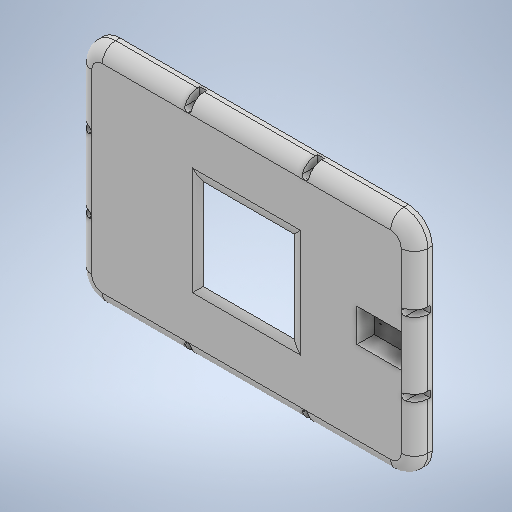
# Autodesk Inventor part: up
Saved by Autodesk Inventor 2025 (Build 290162000, 162)
## iProperties
Created: 2025-10-21
Part Number: up
Material: Generic
Document SubType Name: Modeling
Designer: hp
Density: 1 g/cm^3
Appearance: Default
Author: hp
Autodesk Inventor part; units mm, degrees
ref_plane "YZ Plane" through (0, 0, 0) normal (1, 0, 0) x (0, 1, 0)
ref_plane "XZ Plane" through (0, 0, 0) normal (0, 1, 0) x (-1, 0, 0)
ref_plane "XY Plane" through (0, 0, 0) normal (0, 0, 1) x (1, 0, 0)
sketch "Sketch1" plane through (0, 0, 0) normal (0, 0, 1) x (1, 0, 0)
  line L0 (-325, 254) -> (325, 254)
  line L1 (379, 200) -> (379, -200)
  line L2 (325, -254) -> (-325, -254)
  line L3 (-379, -200) -> (-379, 200)
  line L4 (-379, 254) -> (379, -254) construction
  line L5 (379, 254) -> (-379, -254) construction
  arc A0 (-325, 254) -> (-379, 200) centre (-325, 200) ccw
  arc A1 (379, 200) -> (325, 254) centre (325, 200) ccw
  arc A2 (325, -254) -> (379, -200) centre (325, -200) ccw
  arc A3 (-379, -200) -> (-325, -254) centre (-325, -200) ccw
  point P0 (0, 0)
  dimension "d0" = 758
  dimension "d1" = 508
  dimension "d2" = 54
  constraints: 12 end point, 8 point on circle, 8 point on line, 8 tangent, 4 centre point, 3 equal radius, 2 midpoint, 2 parallel, 1 horizontal, 1 perpendicular
  measures "d0" distance of L4.end L5.end
  measures "d1" distance of L5.start L4.end
  measures "d2" radius of A0
extrude "Extrusion1" add sketch "Sketch1" along normal blind 40
fillet "Fillet1" radius 30 8 edges at (-363.1838, 238.1838, 40) (-379, 0, 40) (-363.1838, -238.1838, 40) (0, -254, 40) (363.1838, -238.1838, 40) (379, 0, 40) (363.1838, 238.1838, 40) (0, 254, 40)
sketch "Sketch2" plane through (0, 0, 0) normal (0, 0, -1) x (-1, 0, 0)
  line L0 (289, 224) -> (-289, 224)
  line L1 (-349, 164) -> (-349, -164)
  line L2 (-289, -224) -> (289, -224)
  line L3 (349, -164) -> (349, 164)
  line L4 (349, 224) -> (-349, -224) construction
  line L5 (-349, 224) -> (349, -224) construction
  arc A0 (349, 164) -> (289, 224) centre (289, 164) ccw
  arc A1 (289, -224) -> (349, -164) centre (289, -164) ccw
  arc A2 (-349, -164) -> (-289, -224) centre (-289, -164) ccw
  arc A3 (-289, 224) -> (-349, 164) centre (-289, 164) ccw
  point P0 (0, 0)
  dimension "d6" = 698
  dimension "d7" = 448
  dimension "d8" = 60
  constraints: 12 end point, 8 point on circle, 8 point on line, 8 tangent, 4 centre point, 3 equal radius, 2 midpoint, 2 parallel, 1 horizontal, 1 perpendicular
  measures "d6" distance of L5.end L4.end
  measures "d7" distance of L5.end L4.start
  measures "d8" radius of A0
extrude "Extrusion2" cut sketch "Sketch2" against normal blind 35
sketch "Sketch3" plane through (0, 0, 40) normal (0, 0, 1) x (1, 0, 0)
  line L0 (-377.7666, 254) -> (272.2334, 254)
  line L1 (-140, 254) -> (-125, 254)
  line L2 (-125, -254) -> (-140, -254)
  line L3 (125, 254) -> (140, 254)
  line L4 (140, -254) -> (125, -254)
  line L5 (-379, -196) -> (-379, 204)
  line L6 (379, 86) -> (379, 71)
  line L7 (-379, 71) -> (-379, 86)
  line L8 (379, 224.0745) -> (379, -175.9255)
  line L9 (379, -79) -> (379, -94)
  line L10 (264.2334, -254) -> (-385.7666, -254)
  line L11 (125, 232.5) -> (125, 254)
  line L12 (140, 254) -> (140, 232.5)
  line L13 (-125, 254) -> (-125, 232.5)
  line L14 (-140, 232.5) -> (-140, 254)
  line L15 (-379, 86) -> (-357.5, 86)
  line L16 (-357.5, 71) -> (-379, 71)
  line L17 (-379, -79) -> (-357.5, -79)
  line L18 (-357.5, -94) -> (-435.7666, -94)
  line L19 (-140, -254) -> (-140, -232.5)
  line L20 (-125, -232.5) -> (-125, -254)
  line L21 (140, -232.5) -> (140, -254)
  line L22 (125, -254) -> (125, -232.5)
  line L23 (357.5, -79) -> (379, -79)
  line L24 (379, -94) -> (357.5, -94)
  line L25 (357.5, 86) -> (379, 86)
  line L26 (379, 71) -> (357.5, 71)
  arc A0 (-140, 232.5) -> (-125, 232.5) centre (-132.5, 232.5) ccw
  arc A1 (125, 232.5) -> (140, 232.5) centre (132.5, 232.5) ccw
  arc A2 (-357.5, 71) -> (-357.5, 86) centre (-357.5, 78.5) ccw
  arc A3 (-357.5, -94) -> (-357.5, -79) centre (-357.5, -86.5) ccw
  arc A4 (-125, -232.5) -> (-140, -232.5) centre (-132.5, -232.5) ccw
  arc A5 (140, -232.5) -> (125, -232.5) centre (132.5, -232.5) ccw
  arc A6 (357.5, -79) -> (357.5, -94) centre (357.5, -86.5) ccw
  arc A7 (357.5, 86) -> (357.5, 71) centre (357.5, 78.5) ccw
  circle A8 centre (132.5, 232.5) radius 2.5
  circle A9 centre (-132.5, 232.5) radius 2.5
  circle A10 centre (-357.5, 78.5) radius 2.5
  circle A11 centre (-357.5, -86.5) radius 2.5
  circle A12 centre (-132.5, -232.5) radius 2.5
  circle A13 centre (132.5, -232.5) radius 2.5
  circle A14 centre (357.5, -86.5) radius 2.5
  circle A15 centre (357.5, 78.5) radius 2.5
  line L27 (325, 254) -> (-325, 254) projected
  line L28 (-325, -254) -> (325, -254) projected
  line L29 (379, -200) -> (379, 200) projected
  line L30 (-379, 200) -> (-379, -200) projected
  line L31 (-102.5, -102.5) -> (102.5, -102.5)
  line L32 (102.5, -102.5) -> (102.5, 102.5)
  line L33 (102.5, 102.5) -> (-102.5, 102.5)
  line L34 (-102.5, 102.5) -> (-102.5, -102.5)
  line L35 (-102.5, -102.5) -> (102.5, 102.5) construction
  line L36 (102.5, -102.5) -> (-102.5, 102.5) construction
  point P0 (0, 0)
  point P1 (-132.5, -254)
  point P2 (132.5, -254)
  point P3 (-423.2666, 71)
  point P4 (301.7334, -79)
  point P5 (301.7334, 71)
  point P6 (301.7334, -94)
  point P7 (125, -163.4255)
  point P8 (-140, -163.4255)
  point P9 (-379, 78.5)
  point P10 (-132.5, -225)
  point P11 (379, -86.5)
  point P12 (-379, -94)
  dimension "d11" = 758
  dimension "d12" = 15
  dimension "d13" = 0
  dimension "d14" = 250
  dimension "d15" = 239
  dimension "d16" = 15
  dimension "d17" = 15
  dimension "d18" = 150
  dimension "d19" = 160
  dimension "d20" = 15
  dimension "d21" = 150
  dimension "d22" = 160
  dimension "d23" = 15
  dimension "d24" = 15
  dimension "d25" = 254
  dimension "d26" = 250
  dimension "d27" = 15
  dimension "d28" = 5
  dimension "d29" = 5
  dimension "d30" = 5
  dimension "d31" = 5
  dimension "d32" = 5
  dimension "d33" = 5
  dimension "d34" = 5
  dimension "d35" = 5
  dimension "d36" = 21.5
  dimension "d37" = 21.5
  dimension "d38" = 21.5
  dimension "d39" = 15
  dimension "d40" = 21.5
  dimension "d41" = 21.5
  dimension "d42" = 29
  dimension "d43" = 21.5
  dimension "d44" = 21.5
  dimension "d83" = 205
  dimension "d84" = 205
  dimension "d87" = 150
  constraints: 66 end point, 21 parallel, 17 point on circle, 16 centre point, 16 tangent, 12 point on line, 9 perpendicular, 8 coincident, 7 horizontal, 6 midpoint, 5 collinear
  measures "d11" distance of L15.start L6.start
  measures "d12" distance of L6.start L6.end
  measures "d13" distance from line of L10 point (-132.5, -254)
  measures "d14" distance from line of L3.start L13
  measures "d15" distance between parallel lines of L8 L12
  measures "d16" distance from line of L3.end L11
  measures "d17" distance between parallel lines of L16 L15
  measures "d18" distance from line of L17 point (-423.267, 71)
  measures "d19" distance between parallel lines of L10 L18
  measures "d20" distance between parallel lines of L18 L17
  measures "d21" distance of point (301.733, -79) point (301.733, 71)
  measures "d22" distance from line of L10 point (301.733, -94)
  measures "d23" distance between parallel lines of L24 L23
  measures "d24" distance from line of point (125, -163.426) L21
  measures "d25" distance from line of L8 point (125, -163.426)
  measures "d26" distance between parallel lines of L22 L20
  measures "d27" distance from line of L20 point (-140, -163.426)
  measures "d28" diameter of A8
  measures "d29" diameter of A9
  measures "d30" diameter of A10
  measures "d31" diameter of A11
  measures "d32" diameter of A12
  measures "d33" diameter of A13
  measures "d34" diameter of A14
  measures "d35" diameter of A15
  measures "d36" distance from line of L4 A5.centre
  measures "d37" distance from line of A1.centre L3
  measures "d38" distance from line of A0.centre L0
  measures "d39" distance between parallel lines of L13 L14
  measures "d40" distance of point (-379, 78.5) A2.centre
  measures "d41" distance from line of L5 A3.centre
  measures "d42" distance from line of L10 point (-132.5, -225)
  measures "d43" distance of point (379, -86.5) A6.centre
  measures "d44" distance from line of A7.centre L6
  measures "d83" distance of L33.end L32.end
  measures "d84" distance of L32.end L31.end
  measures "d87" distance between parallel lines of L23 L26
sketch "Sketch4" plane through (0, 0, 0) normal (0, 0, -1) x (-1, 0, 0)
  line L0 (-329.5439, 254) -> (320.4561, 254)
  line L1 (-140, 254) -> (-125, 254)
  line L2 (-125, -254) -> (-140, -254)
  line L3 (125, 254) -> (140, 254)
  line L4 (140, -254) -> (125, -254)
  line L5 (-379, -204) -> (-379, 196)
  line L6 (379, 86) -> (379, 71)
  line L7 (-379, 71) -> (-379, 86)
  line L8 (379, 206.0747) -> (379, -193.9253)
  line L9 (379, -79) -> (379, -94)
  line L10 (328.4561, -254) -> (-321.5439, -254)
  line L11 (125, 232.5) -> (125, 254)
  line L12 (140, 254) -> (140, 232.5)
  line L13 (-125, 254) -> (-125, 232.5)
  line L14 (-140, 232.5) -> (-140, 254)
  line L15 (-379, 86) -> (-357.5, 86)
  line L16 (-357.5, 71) -> (-379, 71)
  line L17 (-379, -79) -> (-357.5, -79)
  line L18 (-357.5, -94) -> (-371.5439, -94)
  line L19 (-140, -254) -> (-140, -232.5)
  line L20 (-125, -232.5) -> (-125, -254)
  line L21 (140, -232.5) -> (140, -254)
  line L22 (125, -254) -> (125, -232.5)
  line L23 (357.5, -79) -> (379, -79)
  line L24 (379, -94) -> (357.5, -94)
  line L25 (357.5, 86) -> (379, 86)
  line L26 (379, 71) -> (357.5, 71)
  arc A0 (-140, 232.5) -> (-125, 232.5) centre (-132.5, 232.5) ccw
  arc A1 (125, 232.5) -> (140, 232.5) centre (132.5, 232.5) ccw
  arc A2 (-357.5, 71) -> (-357.5, 86) centre (-357.5, 78.5) ccw
  arc A3 (-357.5, -94) -> (-357.5, -79) centre (-357.5, -86.5) ccw
  arc A4 (-125, -232.5) -> (-140, -232.5) centre (-132.5, -232.5) ccw
  arc A5 (140, -232.5) -> (125, -232.5) centre (132.5, -232.5) ccw
  arc A6 (357.5, -79) -> (357.5, -94) centre (357.5, -86.5) ccw
  arc A7 (357.5, 86) -> (357.5, 71) centre (357.5, 78.5) ccw
  circle A8 centre (132.5, 232.5) radius 2.5
  circle A9 centre (-132.5, 232.5) radius 2.5
  circle A10 centre (-357.5, 78.5) radius 2.5
  circle A11 centre (-357.5, -86.5) radius 2.5
  circle A12 centre (-132.5, -232.5) radius 2.5
  circle A13 centre (132.5, -232.5) radius 2.5
  circle A14 centre (357.5, -86.5) radius 2.5
  circle A15 centre (357.5, 78.5) radius 2.5
  line L27 (325, -254) -> (-325, -254) projected
  line L28 (379, 200) -> (379, -200) projected
  line L29 (-379, -200) -> (-379, 200) projected
  line L30 (-325, 254) -> (325, 254) projected
  point P0 (0, 0)
  point P1 (-132.5, -254)
  point P2 (132.5, -254)
  point P3 (-359.0439, 71)
  point P4 (365.9561, -79)
  point P5 (365.9561, 71)
  point P6 (365.9561, -94)
  point P7 (125, -181.4253)
  point P8 (-140, -181.4253)
  point P9 (-379, 78.5)
  point P10 (-132.5, -225)
  point P11 (379, -86.5)
  dimension "d45" = 758
  dimension "d46" = 15
  dimension "d47" = 0
  dimension "d48" = 250
  dimension "d49" = 239
  dimension "d50" = 15
  dimension "d51" = 15
  dimension "d52" = 150
  dimension "d53" = 160
  dimension "d54" = 15
  dimension "d55" = 150
  dimension "d56" = 160
  dimension "d57" = 15
  dimension "d58" = 15
  dimension "d59" = 254
  dimension "d60" = 250
  dimension "d61" = 15
  dimension "d62" = 5
  dimension "d63" = 5
  dimension "d64" = 5
  dimension "d65" = 5
  dimension "d66" = 5
  dimension "d67" = 5
  dimension "d68" = 5
  dimension "d69" = 5
  dimension "d70" = 21.5
  dimension "d71" = 21.5
  dimension "d72" = 21.5
  dimension "d73" = 15
  dimension "d74" = 21.5
  dimension "d75" = 21.5
  dimension "d76" = 29
  dimension "d77" = 21.5
  dimension "d78" = 21.5
  constraints: 54 end point, 19 parallel, 17 point on circle, 16 centre point, 16 tangent, 12 point on line, 8 coincident, 8 perpendicular, 6 horizontal, 5 collinear, 4 midpoint
  measures "d45" distance of L15.start L25.end
  measures "d46" distance of L25.end L6.end
  measures "d47" distance from line of L10 point (-132.5, -254)
  measures "d48" distance from line of L3.start L13
  measures "d49" distance between parallel lines of L8 L12
  measures "d50" distance from line of L12.start L11
  measures "d51" distance between parallel lines of L16 L15
  measures "d52" distance from line of L17 point (-359.044, 71)
  measures "d53" distance between parallel lines of L10 L18
  measures "d54" distance between parallel lines of L18 L17
  measures "d55" distance of point (365.956, -79) point (365.956, 71)
  measures "d56" distance from line of L10 point (365.956, -94)
  measures "d57" distance between parallel lines of L24 L23
  measures "d58" distance from line of point (125, -181.425) L21
  measures "d59" distance from line of L8 point (125, -181.425)
  measures "d60" distance between parallel lines of L22 L20
  measures "d61" distance from line of L20 point (-140, -181.425)
  measures "d62" diameter of A8
  measures "d63" diameter of A9
  measures "d64" diameter of A10
  measures "d65" diameter of A11
  measures "d66" diameter of A12
  measures "d67" diameter of A13
  measures "d68" diameter of A14
  measures "d69" diameter of A15
  measures "d70" distance from line of L4 A5.centre
  measures "d71" distance from line of A1.centre L3
  measures "d72" distance from line of A0.centre L0
  measures "d73" distance between parallel lines of L13 L14
  measures "d74" distance of point (-379, 78.5) A2.centre
  measures "d75" distance from line of L5 A3.centre
  measures "d76" distance from line of L10 point (-132.5, -225)
  measures "d77" distance of point (379, -86.5) A6.centre
  measures "d78" distance from line of A7.centre L6
extrude "Extrusion3" cut sketch "Sketch3" against normal blind 35 contours L0 L13 A0 L14 | L0 L12 A1 L11 | L2 L19 A4 L20 | L4 L22 A5 L21 | L5 L15 A2 L16 | L5 L17 A3 L18 | L6 L26 A7 L25 | L8 L24 A6 L23 | A13
extrude "Extrusion4" cut sketch "Sketch3" against normal through all contours A8 | A9 | A10 | A11 | A12 | A13 | A14 | A15
extrude "Extrusion5" cut sketch "Sketch3" against normal blind 10 contours L34 L33 L32 L31
fillet "Fillet2" radius 40 4 edges at (102.5, 0, 40) (0, -102.5, 40) (-102.5, 0, 40) (0, 102.5, 40)
sketch "Sketch6" plane through (0, 0, 40) normal (0, 0, 1) x (1, 0, 0)
  line L0 (-325, 224) -> (325, 224) projected
  line L1 (283.7823, 13.3743) -> (328.5995, 13.3743)
  line L2 (337.9658, 20.6774) -> (276.5853, 20.6774)
  line L3 (337.9658, 20.6774) -> (276.5853, 20.6774)
  arc A0 (339.1694, 33.055) -> (273.3647, 25.3501) centre (315.2399, -47.431) ccw
  arc A1 (339.1694, 33.055) -> (273.3647, 25.3501) centre (315.2399, -47.431) ccw
  arc A2 (336.6026, 29.0932) -> (276.5202, 21.4818) centre (315.2559, -43.3443) ccw
  arc A3 (336.6026, 29.0932) -> (276.5202, 21.4818) centre (315.2559, -43.3443) ccw
  line L4 (283.7823, 13.3743) -> (328.5995, 13.3743)
  line L5 (337.9658, -19.3226) -> (337.9658, -23.873)
  line L6 (337.9658, 25.2279) -> (337.9658, 20.6774)
  line L7 (337.9658, 25.2279) -> (337.9658, 20.6774)
  line L8 (337.9658, -19.3226) -> (337.9658, -23.873)
  arc A4 (336.6026, 29.0932) -> (337.9658, 25.2279) centre (341.5853, 28.6774) ccw
  arc A5 (337.9658, 25.2279) -> (345.8797, 26.1166) centre (341.5853, 28.6774) ccw
  circle A6 centre (341.5853, 28.6774) radius 2.6
  arc A7 (345.8455, -24.7052) -> (345.8797, 26.1166) centre (244.5247, 0.7738) ccw
  line L9 (328.5995, 13.3743) -> (328.5995, -11.7233)
  line L10 (283.7823, -11.7233) -> (283.7823, 13.3743)
  line L11 (328.5995, 13.3743) -> (328.5995, -11.7233)
  arc A8 (266.5894, 20.4761) -> (266.5894, -19.1212) centre (270.1885, 0.6774) ccw
  line L12 (328.5995, -11.7233) -> (283.7823, -11.7233)
  line L13 (328.5995, -11.7233) -> (283.7823, -11.7233)
  line L14 (276.5853, -19.3226) -> (337.9658, -19.3226)
  line L15 (276.5853, -19.3226) -> (337.9658, -19.3226)
  arc A9 (276.5439, -19.9643) -> (336.5926, -27.592) centre (318.3549, 69.0112) ccw
  arc A10 (276.5439, -19.9643) -> (336.5926, -27.592) centre (318.3549, 69.0112) ccw
  arc A11 (273.3471, -24.0019) -> (339.2228, -31.7292) centre (315.1175, 47.4314) ccw
  arc A12 (273.3471, -24.0019) -> (339.2228, -31.7292) centre (315.1175, 47.4314) ccw
  circle A13 centre (341.5853, 28.6774) radius 2.6
  circle A14 centre (343.2402, 16.9907) radius 1.5
  arc A15 (345.8797, 26.1166) -> (339.1694, 33.055) centre (341.5853, 28.6774) ccw
  circle A16 centre (343.2402, 16.9907) radius 1.5
  circle A17 centre (343.5969, -11.7233) radius 1.5
  circle A18 centre (341.5853, -27.3226) radius 2.6
  circle A19 centre (341.5853, -27.3226) radius 2.6
  circle A20 centre (263.5183, -9.7117) radius 1.5
  circle A21 centre (263.5183, -9.7117) radius 1.5
  circle A22 centre (264.1372, 12.2943) radius 1.5
  circle A23 centre (264.1372, 12.2943) radius 1.5
  circle A24 centre (271.5853, 20.6774) radius 2.6
  line L16 (283.7823, -11.7233) -> (283.7823, 13.3743)
  circle A25 centre (271.5853, 20.6774) radius 2.6
  circle A26 centre (271.5853, -19.3226) radius 2.6
  circle A27 centre (271.5853, -19.3226) radius 2.6
  arc A28 (266.5894, 20.4761) -> (266.5894, -19.1212) centre (270.1885, 0.6774) ccw
  arc A29 (339.1694, 33.055) -> (336.6026, 29.0932) centre (341.5853, 28.6774) ccw
  arc A30 (345.8455, -24.7052) -> (345.8797, 26.1166) centre (244.5247, 0.7738) ccw
  circle A31 centre (341.5853, 28.6774) radius 5
  circle A32 centre (271.5853, 20.6774) radius 5
  arc A33 (266.5894, 20.4761) -> (276.5853, 20.6774) centre (271.5853, 20.6774) ccw
  arc A34 (276.5853, 20.6774) -> (276.5202, 21.4818) centre (271.5853, 20.6774) ccw
  arc A35 (276.5202, 21.4818) -> (273.3647, 25.3501) centre (271.5853, 20.6774) ccw
  arc A36 (273.3647, 25.3501) -> (266.5894, 20.4761) centre (271.5853, 20.6774) ccw
  circle A37 centre (271.5853, -19.3226) radius 5
  circle A38 centre (343.5969, -11.7233) radius 1.5
  arc A39 (336.5926, -27.592) -> (339.2228, -31.7292) centre (341.5853, -27.3226) ccw
  arc A40 (345.8455, -24.7052) -> (337.9658, -23.873) centre (341.5853, -27.3226) ccw
  circle A41 centre (341.5853, -27.3226) radius 5
  arc A42 (339.2228, -31.7292) -> (345.8455, -24.7052) centre (341.5853, -27.3226) ccw
  arc A43 (337.9658, -23.873) -> (336.5926, -27.592) centre (341.5853, -27.3226) ccw
  arc A44 (276.5439, -19.9643) -> (276.5853, -19.3226) centre (271.5853, -19.3226) ccw
  arc A45 (273.3471, -24.0019) -> (276.5439, -19.9643) centre (271.5853, -19.3226) ccw
  arc A46 (266.5894, -19.1212) -> (273.3471, -24.0019) centre (271.5853, -19.3226) ccw
  arc A47 (276.5853, -19.3226) -> (266.5894, -19.1212) centre (271.5853, -19.3226) ccw
  line L17 (349, 200) -> (349, -200) projected
  line L18 (325, -224) -> (-325, -224) projected
  line L19 (349, 37.5) -> (249, 37.5)
  line L20 (249, 37.5) -> (249, -37.5)
  line L21 (249, -37.5) -> (349, -37.5)
  line L22 (349, -37.5) -> (349, 37.5)
  line L23 (245, -41.5) -> (245, 41.5)
  line L24 (245, 41.5) -> (353, 41.5)
  line L25 (353, 41.5) -> (353, -41.5)
  line L26 (353, -41.5) -> (245, -41.5)
  point P0 (0, 0)
  point P1 (349, 41.5)
  point P2 (349, -41.5)
  dimension "d4" = 0
  dimension "d7" = 448
  dimension "d106" = 3
  dimension "d107" = 5
  dimension "d108" = 5.2
  dimension "d109" = 98.3096
  dimension "d110" = 75.5173
  dimension "d111" = 83.968
  dimension "d112" = 82.7495
  dimension "d113" = 20.1231
  dimension "d114" = 104.4753
  dimension "d115" = 0
  dimension "d116" = 9.3663
  dimension "d117" = 54.1835
  dimension "d118" = 32.4008
  dimension "d119" = 7.3031
  dimension "d120" = 40
  dimension "d121" = 7.9139
  dimension "d122" = 5.4391
  dimension "d123" = 7.8797
  dimension "d124" = 45.3826
  dimension "d125" = 5.6311
  dimension "d126" = 32.4008
  dimension "d127" = 5.2744
  dimension "d128" = 3.6867
  dimension "d129" = 3.6195
  dimension "d130" = 3.6195
  dimension "d131" = 1.257
  dimension "d132" = 1.2036
  dimension "d133" = 1.3632
  dimension "d134" = 1.3733
  dimension "d135" = 19.611
  dimension "d136" = 22.7099
  dimension "d137" = 22.7259
  dimension "d138" = 22.8483
  dimension "d139" = 61.3805
  dimension "d140" = 61.3805
  dimension "d141" = 61.4219
  dimension "d142" = 61.4456
  dimension "d143" = 67.7774
  dimension "d144" = 20
  dimension "d145" = 73.8286
  dimension "d146" = 8.3831
  dimension "d147" = 74.4475
  dimension "d148" = 30.3891
  dimension "d149" = 271.431
  dimension "d152" = 271.4314
  dimension "d153" = 25.0977
  dimension "d154" = 75
  dimension "d155" = 186.5
  dimension "d156" = 100
  dimension "d159" = 4
  constraints: 56 point on circle, 48 centre point, 48 end point, 31 tangent, 24 concentric, 9 equal radius, 6 parallel, 6 perpendicular, 1 collinear, 1 horizontal, 1 point on line, 3 other
  measures "d106" diameter of A38
  measures "d107" radius of A5
  measures "d108" diameter of A6
  measures "d109" radius of A10
  measures "d110" radius of A3
  measures "d111" radius of A1
  measures "d112" radius of A12
  measures "d113" radius of A28
  measures "d114" radius of A30
  measures "d115" distance between parallel lines of L5 L6
  measures "d116" distance between parallel lines of L11 L6
  measures "d117" distance between parallel lines of L16 L6
  measures "d118" distance between parallel lines of L12 L3
  measures "d119" distance between parallel lines of L1 L3
  measures "d120" distance between parallel lines of L14 L3
  measures "d121" distance from line of A5.end L6
  measures "d122" distance from line of A5.end L3
  measures "d123" distance from line of A7.start L6
  measures "d124" distance from line of A7.start L3
  measures "d125" distance from line of A38.centre L6
  measures "d126" distance from line of A38.centre L3
  measures "d127" distance from line of A14.centre L6
  measures "d128" distance from line of A14.centre L3
  measures "d129" distance from line of A5.centre L6
  measures "d130" distance from line of A43.centre L6
  measures "d131" distance from line of A11.end L6
  measures "d132" distance from line of A0.start L6
  measures "d133" distance from line of A2.start L6
  measures "d134" distance from line of A9.end L6
  measures "d135" distance from line of A10.centre L6
  measures "d136" distance from line of A3.centre L6
  measures "d137" distance from line of A1.centre L6
  measures "d138" distance from line of A12.centre L6
  measures "d139" distance from line of L2.end L6
  measures "d140" distance from line of L14.start L6
  measures "d141" distance from line of A9.start L6
  measures "d142" distance from line of A2.end L6
  measures "d143" distance from line of A28.centre L6
  measures "d144" distance from line of A28.centre L3
  measures "d145" distance from line of A23.centre L6
  measures "d146" distance from line of A23.centre L3
  measures "d147" distance from line of A20.centre L6
  measures "d148" distance from line of A20.centre L3
  measures "d149" distance from line of L0 A0.centre
  measures "d152" distance from line of L18 A11.centre
  measures "d153" distance between parallel lines of L1 L12
  measures "d154" distance of L19.end L20.end
  measures "d155" distance between parallel lines of L0 L19
  measures "d156" distance between parallel lines of L22 L20
  measures "d159" distance between parallel lines of L20 L23
extrude "Extrusion6" cut sketch "Sketch6" against normal blind 15.24 contours L1 L9 L12 L10 | L6 A5 A7 A40 L5 L14 A37 A8 A32 L2 | L2 A32 A2 A4 L6 | A32 | A4 A29 A15 A5 | A32 A0 A29 A2 | L17 L21 L20 L19 | A37 | L14 L5 A41 A9 A37 | A37 A9 A39 A11 | A41 A39 A40 | L19 L20 L21 L17 L26 L23 L24 | A6 | A14 | A17 | A18 | A20 | A22 | A24 | A26
extrude "Extrusion7" add sketch "Sketch6" against normal blind 43.12 contours L19 L20 L21 L17 L26 L23 L24
extrude "Extrusion8" add sketch "Sketch6" against normal blind 43.12 contours L1 L9 L12 L10 | L6 A5 A7 A40 L5 L14 A37 A8 A32 L2 | L2 A32 A2 A4 L6 | A32 | A4 A29 A15 A5 | A32 A0 A29 A2 | L17 L21 L20 L19 | A37 | L14 L5 A41 A9 A37 | A37 A9 A39 A11 | A41 A39 A40 | A6 | A14 | A17 | A18 | A20 | A22 | A24 | A26
extrude "Extrusion9" cut sketch "Sketch6" against normal blind 39.12 contours L1 L9 L12 L10 | L6 A5 A7 A40 L5 L14 A37 A8 A32 L2 | L2 A32 A2 A4 L6 | A32 | A4 A29 A15 A5 | A32 A0 A29 A2 | L17 L21 L20 L19 | A37 | L14 L5 A41 A9 A37 | A37 A9 A39 A11 | A41 A39 A40 | A6 | A14 | A17 | A18 | A20 | A22 | A24 | A26
extrude "Extrusion10" cut sketch "Sketch6" against normal through all contours A14 | A17 | A20 | A22
body "Solid1"
